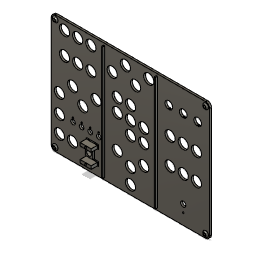
CP-BO Front v3 (Autodesk Fusion 360 design; units mm, degrees)
Autodesk Fusion 360 part; units mm, degrees
note: some values were not read from the file. Set by a fixed rule: which sketch regions a step uses.
sketch "Esquisse1" plane through (0, 0, 0) normal (0, 0, 1) x (1, 0, 0)
  line L0 (10, 0) -> (255, 0)
  line L1 (265, 10) -> (265, 190)
  line L2 (255, 200) -> (10, 200)
  line L3 (0, 190) -> (0, 10)
  arc A0 (10, 200) -> (0, 190) centre (10, 190) ccw
  arc A1 (265, 190) -> (255, 200) centre (255, 190) ccw
  arc A2 (255, 0) -> (265, 10) centre (255, 10) ccw
  arc A3 (0, 10) -> (10, 0) centre (10, 10) ccw
  line L4 (3.6, 190) -> (3.6, 10)
  arc A4 (3.6, 10) -> (10, 3.6) centre (10, 10) ccw
  line L5 (10, 3.6) -> (255, 3.6)
  arc A5 (255, 3.6) -> (261.4, 10) centre (255, 10) ccw
  line L6 (261.4, 10) -> (261.4, 190)
  arc A6 (261.4, 190) -> (255, 196.4) centre (255, 190) ccw
  line L7 (255, 196.4) -> (10, 196.4)
  arc A7 (10, 196.4) -> (3.6, 190) centre (10, 190) ccw
  circle A8 centre (10, 190) radius 1.6
  circle A9 centre (10, 190) radius 2.6
  circle A10 centre (10, 190) radius 3.5
  circle A11 centre (255, 190) radius 1.6
  circle A12 centre (255, 190) radius 2.6
  circle A13 centre (255, 190) radius 3.5
  circle A14 centre (10, 10) radius 1.6
  circle A15 centre (10, 10) radius 2.6
  circle A16 centre (10, 10) radius 3.5
  circle A17 centre (255, 10) radius 1.6
  circle A18 centre (255, 10) radius 2.6
  circle A19 centre (255, 10) radius 3.5
  point P0 (265, 0)
  point P1 (0, 200)
  dimension "d1" = 265
  dimension "d2" = 200
  dimension "d3" = 10
  dimension "d4" = -3.6
  dimension "d5" = 3.2
  dimension "d6" = 5.2
  dimension "d7" = 7
  dimension "d10" = 245
  dimension "d11" = -180
  constraint horizontal L0
  constraint vertical L1
  constraint horizontal L2
  constraint vertical L3
  constraint coincident P1 L2
  constraint coincident P1 L3
  constraint tangent L2 A0
  constraint tangent L3 A0
  constraint tangent L1 A1
  constraint tangent L2 A1
  constraint equal A0 A1
  constraint coincident P0 L0
  constraint coincident P0 L1
  constraint tangent L0 A2
  constraint tangent L1 A2
  constraint equal A0 A2
  constraint coincident origin L0
  constraint coincident origin L3
  constraint tangent L0 A3
  constraint tangent L3 A3
  constraint equal A0 A3
  constraint concentric A0 A8
  constraint concentric A0 A9
  constraint concentric A0 A10
  measures "d1" distance of origin P0
  measures "d2" distance of origin P1
  measures "d3" radius of A0
  measures "d5" diameter of A8
  measures "d6" diameter of A9
  measures "d7" diameter of A10
extrude "Extrusion1" add sketch "Esquisse1" along normal blind 3 contours L4 A4 L5 A5 L6 A6 L7 A7
extrude "Extrusion2" add sketch "Esquisse1" along normal blind 3 and the other way blind -2 contours A9 | A10 | A12 | A13 | A15 | A16 | A18 | A19
extrude "Extrusion3" add sketch "Esquisse1" along normal blind 5 and the other way blind -2 contours A9 | A12 | A15 | A18
fillet "Congé1" radius 2 4 edges at (252.5759, 10.9402, 3) (7.5759, 10.9402, 3) (7.5759, 190.9402, 3) (252.5759, 190.9402, 3)
sketch "Esquisse2" plane through (0, 0, 3) normal (0, 0, 1) x (1, 0, 0)
  circle A0 centre (10, 190) radius 4.6
  circle A1 centre (255, 10) radius 4.6
  arc A2 (10, 196.4) -> (3.6, 190) centre (10, 190) ccw
  line L0 (3.6, 190) -> (3.6, 10)
  arc A3 (3.6, 10) -> (10, 3.6) centre (10, 10) ccw
  line L1 (10, 3.6) -> (255, 3.6)
  arc A4 (255, 3.6) -> (261.4, 10) centre (255, 10) ccw
  line L2 (261.4, 10) -> (261.4, 190)
  arc A5 (261.4, 190) -> (255, 196.4) centre (255, 190) ccw
  line L3 (255, 196.4) -> (10, 196.4)
  circle A6 centre (10, 10) radius 4.6
  circle A7 centre (255, 190) radius 4.6
  line L4 (89.5333, 196.4) -> (89.5333, 3.6) construction
  line L5 (175.4667, 196.4) -> (175.4667, 3.6) construction
  line L6 (175.4667, 33.6) -> (261.4, 33.6) construction
  line L7 (175.4667, 76.2) -> (261.4, 76.2) construction
  line L8 (175.4667, 118.8) -> (261.4, 118.8) construction
  line L9 (175.4667, 161.4) -> (261.4, 161.4) construction
  line L10 (196.95, 196.4) -> (196.95, 3.6) construction
  line L11 (218.4333, 196.4) -> (218.4333, 3.6) construction
  line L12 (239.9167, 196.4) -> (239.9167, 3.6) construction
  circle A8 centre (218.4333, 33.6) radius 4.2
  circle A9 centre (196.95, 76.2) radius 8.3
  circle A10 centre (218.4333, 76.2) radius 8.3
  circle A11 centre (239.9167, 76.2) radius 8.3
  circle A12 centre (196.95, 118.8) radius 8.3
  circle A13 centre (218.4333, 118.8) radius 8.3
  circle A14 centre (239.9167, 118.8) radius 8.3
  line L13 (188.65, 100) -> (188.65, 105) construction
  line L14 (188.65, 105) -> (188.65, 196.4) construction
  line L15 (248.2167, 100) -> (248.2167, 196.4) construction
  circle A15 centre (218.4333, 161.4) radius 6.25
  circle A16 centre (194.9, 161.4) radius 6.25
  circle A17 centre (241.9667, 161.4) radius 6.25
  line L16 (89.5333, 18) -> (175.4667, 18) construction
  line L17 (89.5333, 55.2106) -> (175.4667, 55.2106) construction
  line L18 (111.0167, 196.4) -> (111.0167, 3.6) construction
  line L19 (132.5, 196.4) -> (132.5, 3.6) construction
  line L20 (153.9833, 196.4) -> (153.9833, 3.6) construction
  circle A18 centre (111.0167, 55.2106) radius 8.3
  circle A19 centre (153.9833, 55.2106) radius 8.3
  circle A20 centre (132.5, 18) radius 8.3
  circle A21 centre (132.5, 42.8106) radius 8.3
  line L21 (89.5333, 108.6053) -> (175.4667, 108.6053) construction
  line L22 (89.5333, 87.1223) -> (175.4667, 87.1223) construction
  line L23 (89.5333, 130.0883) -> (175.4667, 130.0883) construction
  circle A22 centre (132.5, 108.6053) radius 8.3
  circle A23 centre (153.9833, 108.6053) radius 8.3
  circle A24 centre (111.0167, 108.6053) radius 8.3
  circle A25 centre (132.5, 130.0883) radius 8.3
  circle A26 centre (111.0167, 130.0883) radius 8.3
  circle A27 centre (132.5, 87.1223) radius 8.3
  circle A28 centre (153.9833, 87.1223) radius 8.3
  line L24 (89.5333, 182) -> (175.4667, 182) construction
  line L25 (89.5333, 162) -> (175.4667, 162) construction
  circle A29 centre (162.2833, 182) radius 8.3
  circle A30 centre (140.8, 162) radius 8.3
  circle A31 centre (124.2, 182) radius 8.3
  circle A32 centre (102.7167, 162) radius 8.3
  line L26 (68.05, 196.4) -> (68.05, 3.6) construction
  line L27 (46.5667, 196.4) -> (46.5667, 3.6) construction
  line L28 (25.0833, 196.4) -> (25.0833, 3.6) construction
  line L29 (89.5333, 182) -> (3.6, 182) construction
  line L30 (89.5333, 145.8) -> (3.6, 145.8) construction
  line L31 (89.5333, 109.6) -> (3.6, 109.6) construction
  line L32 (89.5333, 89.6) -> (3.6, 89.6) construction
  line L33 (89.5333, 59.6) -> (3.6, 59.6) construction
  line L34 (89.5333, 31.6) -> (3.6, 31.6) construction
  circle A33 centre (25.0833, 182) radius 8.3
  circle A34 centre (46.5667, 182) radius 8.3
  circle A35 centre (68.05, 182) radius 8.3
  circle A36 centre (25.0833, 145.8) radius 8.3
  circle A37 centre (46.5667, 145.8) radius 8.3
  circle A38 centre (68.05, 145.8) radius 8.3
  circle A39 centre (76.35, 109.6) radius 8.3
  circle A40 centre (38.2667, 109.6) radius 8.3
  circle A41 centre (54.8667, 89.6) radius 8.3
  circle A42 centre (16.7833, 89.6) radius 8.3
  line L35 (16.7833, 108.886) -> (16.7833, 3.6) construction
  circle A43 centre (16.7833, 59.6) radius 8.3
  circle A44 centre (16.7833, 31.6) radius 8.3
  line L36 (39.0375, 69) -> (39.0375, 49) construction
  line L37 (52.9917, 69) -> (52.9917, 49) construction
  line L38 (66.9458, 69) -> (66.9458, 49) construction
  line L39 (80.9, 69) -> (80.9, 48.7369) construction
  circle A45 centre (39.0375, 59.6) radius 3.75
  circle A46 centre (52.9917, 59.6) radius 3.75
  circle A47 centre (66.9458, 59.6) radius 3.75
  circle A48 centre (80.9, 59.6) radius 3.75
  line L40 (84.65, 126.0158) -> (84.65, 39.0422) construction
  line L41 (194.9, 171) -> (194.9, 151) construction
  line L42 (241.9667, 172) -> (241.9667, 151) construction
  line L43 (194.2, 156.2) -> (195.6, 156.2)
  line L44 (195.6, 156.2) -> (195.6, 155.15)
  line L45 (195.6, 155.15) -> (194.2, 155.15)
  line L46 (194.2, 155.15) -> (194.2, 156.2)
  line L47 (217.7333, 156.2) -> (219.1333, 156.2)
  line L48 (219.1333, 156.2) -> (219.1333, 155.15)
  line L49 (219.1333, 155.15) -> (217.7333, 155.15)
  line L50 (217.7333, 155.15) -> (217.7333, 156.2)
  line L51 (241.2667, 156.2) -> (242.6667, 156.2)
  line L52 (242.6667, 156.2) -> (242.6667, 155.15)
  line L53 (242.6667, 155.15) -> (241.2667, 155.15)
  line L54 (241.2667, 155.15) -> (241.2667, 156.2)
  circle A49 centre (218.4333, 21.6) radius 1.3
  line L55 (87, 65.6) -> (36, 65.6) construction
  circle A50 centre (39.0375, 65.6) radius 1.25
  circle A51 centre (52.9917, 65.6) radius 1.25
  circle A52 centre (66.9458, 65.6) radius 1.25
  circle A53 centre (80.9, 65.6) radius 1.25
  circle A54 centre (68.05, 31.6) radius 3.95
  line L56 (38.0624, 123.6693) -> (38.0624, 15) construction
  circle A55 centre (38.0624, 31.6) radius 8.3
  line L57 (88.5333, 192.8) -> (90.5333, 192.8)
  line L58 (90.5333, 192.8) -> (90.5333, 7.2)
  line L59 (90.5333, 7.2) -> (88.5333, 7.2)
  line L60 (88.5333, 7.2) -> (88.5333, 192.8)
  line L61 (174.4667, 192.8) -> (176.4667, 192.8)
  line L62 (176.4667, 192.8) -> (176.4667, 7.2)
  line L63 (176.4667, 7.2) -> (174.4667, 7.2)
  line L64 (174.4667, 7.2) -> (174.4667, 192.8)
  line L65 (57.05, 42.6) -> (84.05, 42.6) construction
  line L66 (84.05, 42.6) -> (84.05, 23.6) construction
  line L67 (84.05, 23.6) -> (57.05, 23.6) construction
  line L68 (57.05, 23.6) -> (57.05, 42.6) construction
  line L69 (61.55, 42.6) -> (79.55, 42.6)
  line L70 (79.55, 42.6) -> (79.55, 47.6)
  line L71 (79.55, 47.6) -> (61.55, 47.6)
  line L72 (61.55, 47.6) -> (61.55, 42.6)
  line L73 (61.55, 23.6) -> (79.55, 23.6)
  line L74 (79.55, 23.6) -> (79.55, 18.6)
  line L75 (79.55, 18.6) -> (61.55, 18.6)
  line L76 (61.55, 18.6) -> (61.55, 23.6)
  line L77 (70.55, 23.6) -> (70.55, 47.6) construction
  line L78 (61.55, 45.1) -> (79.55, 45.1) construction
  line L79 (61.55, 21.1) -> (79.55, 21.1) construction
  circle A56 centre (70.55, 45.1) radius 1.5
  circle A57 centre (70.55, 21.1) radius 1.5
  line L80 (62.05, 37.6) -> (74.05, 37.6)
  line L81 (74.05, 37.6) -> (74.05, 25.6)
  line L82 (74.05, 25.6) -> (62.05, 25.6)
  line L83 (62.05, 25.6) -> (62.05, 37.6)
  dimension "d24" = 30
  dimension "d27" = 35
  dimension "d29" = 8.4
  dimension "d30" = 16.6
  dimension "d31" = 16.6
  dimension "d32" = 16.6
  dimension "d33" = 16.6
  dimension "d34" = 16.6
  dimension "d35" = 16.6
  dimension "d36" = 12.5
  dimension "d37" = 12.5
  dimension "d38" = 12.5
  dimension "d39" = 14.4
  dimension "d40" = 16.6
  dimension "d41" = 16.6
  dimension "d42" = 16.6
  dimension "d43" = 42.967
  dimension "d44" = 16.6
  dimension "d45" = 12.4
  dimension "d46" = 37.2106
  dimension "d47" = 16.6
  dimension "d48" = 16.6
  dimension "d49" = 16.6
  dimension "d50" = 16.6
  dimension "d51" = 16.6
  dimension "d52" = 16.6
  dimension "d53" = 16.6
  dimension "d54" = 21.483
  dimension "d55" = 21.667
  dimension "d56" = 21.4833
  dimension "d57" = 14.4
  dimension "d58" = 16.6
  dimension "d59" = 16.6
  dimension "d60" = 16.6
  dimension "d61" = 16.6
  dimension "d62" = 20
  dimension "d63" = 16.6
  dimension "d64" = 16.6
  dimension "d65" = 16.6
  dimension "d66" = 14.4
  dimension "d67" = 16.6
  dimension "d68" = 16.6
  dimension "d69" = 16.6
  dimension "d70" = 20
  dimension "d71" = 16.6
  dimension "d72" = 16.6
  dimension "d73" = 16.6
  dimension "d74" = 16.6
  dimension "d75" = 16.6
  dimension "d76" = 16.6
  dimension "d77" = 28
  dimension "d78" = 7.5
  dimension "d79" = 7.5
  dimension "d80" = 7.5
  dimension "d81" = 7.5
  dimension "d84" = 28
  dimension "d86" = 30
  dimension "d87" = 32.6492
  dimension "d88" = 1.4
  dimension "d89" = 1.4
  dimension "d90" = 1.4
  dimension "d91" = 5.2
  dimension "d92" = 5.2
  dimension "d93" = 5.2
  dimension "d94" = 2.6
  dimension "d95" = 12
  dimension "d96" = 2.5
  dimension "d97" = 2.5
  dimension "d98" = 2.5
  dimension "d99" = 2.5
  dimension "d100" = 6
  dimension "d101" = 7.9
  dimension "d102" = 16.6
  dimension "d110" = 2
  dimension "d111" = 2
  dimension "d114" = 3.6
  dimension "d115" = 3.6
  dimension "d116" = 3.6
  dimension "d117" = 3.6
  dimension "d126" = 19
  dimension "d127" = 27
  dimension "d128" = 11
  dimension "d129" = 8
  dimension "d130" = 18
  dimension "d131" = 18
  dimension "d132" = 5
  dimension "d133" = 5
  dimension "d134" = 3
  dimension "d135" = 3
  dimension "d136" = 12
  dimension "d137" = 12
  constraint coincident L3 L4.start
  constraint coincident L1 L4.end
  constraint perpendicular L1 L4
  constraint coincident L3 L5.start
  constraint perpendicular L1 L5
  constraint coincident L5 L6.start
  constraint coincident L2 L6.end
  constraint perpendicular L2 L6
  constraint coincident L5 L7.start
  constraint coincident L2 L7.end
  constraint perpendicular L2 L7
  constraint coincident L5 L8.start
  constraint coincident L2 L8.end
  constraint perpendicular L2 L8
  constraint coincident L5 L9.start
  constraint coincident L2 L9.end
  constraint perpendicular L2 L9
  constraint symmetric L7 L8 L9
  constraint symmetric L6 L7 L8
  constraint coincident L3 L10.start
  constraint coincident L1 L10.end
  constraint perpendicular L1 L10
  constraint coincident L3 L11.start
  constraint coincident L1 L11.end
  constraint perpendicular L1 L11
  constraint coincident L1 L12.end
  constraint perpendicular L1 L12
  constraint symmetric L10 L11 L12
  constraint symmetric L5 L10 L11
  constraint coincident L11 A8.centre
  constraint coincident L6 A8.centre
  constraint coincident L7 A9.centre
  constraint coincident L10 A9.centre
  constraint midpoint L7 A10.centre
  constraint coincident L12 A11.centre
  constraint coincident L7 A11.centre
  constraint coincident L10 A12.centre
  constraint coincident L8 A12.centre
  constraint midpoint L8 A13.centre
  constraint coincident L8 A14.centre
  constraint coincident L12 A14.centre
  constraint perpendicular L8 L13
  constraint perpendicular L9 L14
  constraint coincident L3 L15.end
  constraint perpendicular L3 L15
  constraint coincident L3 L14.end
  constraint tangent A12 L14
  constraint tangent A14 L15
  constraint midpoint L9 A15.centre
  constraint coincident L9 A16.centre
  constraint coincident L9 A17.centre
  constraint tangent L14 A16
  constraint tangent L15 A17
  constraint coincident L4 L16.start
  constraint coincident L5 L16.end
  constraint perpendicular L5 L16
  constraint coincident L4 L17.start
  constraint coincident L5 L17.end
  constraint perpendicular L5 L17
  constraint coincident L3 L18.start
  constraint coincident L1 L18.end
  constraint perpendicular L1 L18
  constraint coincident L3 L19.start
  constraint perpendicular L16 L19
  constraint coincident L3 L20.start
  constraint coincident L1 L20.end
  constraint perpendicular L1 L20
  constraint coincident L1 L19.end
  constraint symmetric L5 L19 L20
  constraint symmetric L4 L18 L19
  constraint coincident L18 A18.centre
  constraint coincident L17 A18.centre
  constraint coincident L17 A19.centre
  constraint coincident L20 A19.centre
  constraint midpoint L16 A20.centre
  constraint coincident L19 A21.centre
  constraint coincident L4 L21.start
  constraint coincident L5 L21.end
  constraint coincident L4 L22.start
  constraint coincident L5 L22.end
  constraint perpendicular L5 L22
  constraint coincident L4 L23.start
  constraint coincident L5 L23.end
  constraint perpendicular L5 L23
  constraint midpoint L21 A22.centre
  constraint coincident L21 A23.centre
  constraint coincident L20 A23.centre
  constraint coincident L21 A24.centre
  constraint coincident L18 A24.centre
  constraint midpoint L23 A25.centre
  constraint coincident L23 A26.centre
  constraint coincident L18 A26.centre
  constraint midpoint L22 A27.centre
  constraint coincident L20 A28.centre
  constraint coincident L22 A28.centre
  constraint symmetric L21 L22 L23
  constraint coincident L4 L24.start
  constraint coincident L5 L24.end
  constraint perpendicular L5 L24
  constraint coincident L4 L25.start
  constraint perpendicular L20 L25
  constraint coincident L24 A29.centre
  constraint coincident L25 A30.centre
  constraint coincident L24 A31.centre
  constraint coincident L25 A32.centre
  constraint tangent L20 A29
  constraint tangent L18 A32
  constraint symmetric L17 L21 L25
  constraint tangent L19 A30
  constraint tangent L19 A31
  constraint coincident L3 L26.start
  constraint coincident L1 L26.end
  constraint perpendicular L1 L26
  constraint coincident L3 L27.start
  constraint coincident L1 L27.end
  constraint perpendicular L1 L27
  constraint coincident L3 L28.start
  constraint coincident L1 L28.end
  constraint perpendicular L1 L28
  constraint symmetric L26 L27 L28
  constraint coincident L0 L29.end
  constraint perpendicular L0 L29
  constraint coincident L4 L30.start
  constraint coincident L0 L30.end
  constraint perpendicular L0 L30
  constraint coincident L4 L31.start
  constraint coincident L0 L31.end
  constraint perpendicular L0 L31
  constraint coincident L4 L32.start
  constraint coincident L0 L32.end
  constraint perpendicular L0 L32
  constraint coincident L4 L33.start
  constraint coincident L0 L33.end
  constraint perpendicular L0 L33
  constraint coincident L4 L34.start
  constraint coincident L0 L34.end
  constraint perpendicular L0 L34
  constraint coincident L29 A33.centre
  constraint coincident L28 A33.centre
  constraint midpoint L29 A34.centre
  constraint coincident L29 A35.centre
  constraint coincident L26 A35.centre
  constraint coincident L30 A36.centre
  constraint coincident L28 A36.centre
  constraint midpoint L30 A37.centre
  constraint coincident L30 A38.centre
  constraint coincident L26 A38.centre
  constraint coincident L31 A40.centre
  constraint coincident L32 A41.centre
  constraint coincident L32 A42.centre
  constraint tangent L27 A40
  constraint tangent L26 A39
  constraint tangent L27 A41
  constraint tangent L28 A42
  constraint coincident L1 L35.end
  constraint perpendicular L1 L35
  constraint coincident A42.centre L35
  constraint coincident L35 A43.centre
  constraint coincident L33 A43.centre
  constraint coincident L35 A44.centre
  constraint coincident L34 A44.centre
  constraint perpendicular L33 L36
  constraint perpendicular L33 L37
  constraint perpendicular L33 L38
  constraint perpendicular L33 L39
  constraint symmetric L36 L37 L38
  constraint coincident L36 A45.centre
  constraint coincident L33 A45.centre
  constraint coincident L33 A46.centre
  constraint coincident L33 A47.centre
  constraint coincident L39 A48.centre
  constraint coincident L33 A48.centre
  constraint coincident L37 A46.centre
  constraint coincident L38 A47.centre
  constraint coincident L31 A39.centre
  constraint tangent A48 L40
  constraint tangent A39 L40
  constraint parallel L4 L40
  constraint symmetric L29 L30 L31
  constraint parallel L10 L41
  constraint perpendicular L9 L42
  constraint coincident A17.centre L42
  constraint coincident A16.centre L41
  constraint horizontal L43
  constraint vertical L44
  constraint horizontal L45
  constraint vertical L46
  constraint horizontal L47
  constraint vertical L48
  constraint horizontal L49
  constraint vertical L50
  constraint horizontal L51
  constraint vertical L52
  constraint horizontal L53
  constraint vertical L54
  constraint symmetric L41 L44 L46
  constraint symmetric L11 L48 L50
  constraint symmetric L42 L52 L54
  constraint tangent A16 L45
  constraint tangent A15 L49
  constraint tangent A17 L53
  constraint coincident L11 A49.centre
  constraint perpendicular L36 L55
  constraint coincident L55 A50.centre
  constraint coincident L55 A51.centre
  constraint coincident L55 A52.centre
  constraint coincident L55 A53.centre
  constraint coincident L36 A50.centre
  constraint coincident L37 A51.centre
  constraint coincident L38 A52.centre
  constraint coincident L39 A53.centre
  constraint coincident L34 A54.centre
  constraint coincident L26 A54.centre
  constraint perpendicular L34 L56
  constraint coincident L34 A55.centre
  constraint coincident L56 A55.centre
  constraint horizontal L57
  constraint vertical L58
  constraint horizontal L59
  constraint vertical L60
  constraint horizontal L61
  constraint vertical L62
  constraint horizontal L63
  constraint vertical L64
  constraint symmetric L4 L58 L60
  constraint symmetric L5 L62 L64
  constraint coincident L1 L5.end
  constraint horizontal L65
  constraint vertical L66
  constraint horizontal L67
  constraint vertical L68
  constraint horizontal L69
  constraint vertical L70
  constraint horizontal L71
  constraint vertical L72
  constraint coincident L65 L69.start
  constraint horizontal L73
  constraint vertical L74
  constraint horizontal L75
  constraint vertical L76
  constraint coincident L67 L73.start
  constraint midpoint L67 L77.start
  constraint coincident L71 L77.end
  constraint perpendicular L71 L77
  constraint symmetric L70 L72 L77
  constraint symmetric L74 L76 L77
  constraint midpoint L72 L78.start
  constraint midpoint L70 L78.end
  constraint midpoint L76 L79.start
  constraint midpoint L74 L79.end
  constraint midpoint L78 A56.centre
  constraint midpoint L79 A57.centre
  constraint horizontal L80
  constraint vertical L81
  constraint horizontal L82
  constraint vertical L83
  constraint symmetric L34 L80 L82
  constraint symmetric L26 L81 L83
  measures "d24" distance of L1 L6
  measures "d27" distance of L3 L9
  measures "d29" diameter of A8
  measures "d30" diameter of A9
  measures "d31" diameter of A10
  measures "d32" diameter of A11
  measures "d33" diameter of A12
  measures "d34" diameter of A13
  measures "d35" diameter of A14
  measures "d36" diameter of A15
  measures "d37" diameter of A16
  measures "d38" diameter of A17
  measures "d39" distance of L1 L16
  measures "d40" diameter of A18
  measures "d41" diameter of A19
  measures "d42" diameter of A20
  measures "d43" distance of A19.centre A20.centre
  measures "d44" diameter of A21
  measures "d45" distance of L17 A21.centre
  measures "d46" distance of L16 L17
  measures "d47" diameter of A22
  measures "d48" diameter of A23
  measures "d49" diameter of A24
  measures "d50" diameter of A25
  measures "d51" diameter of A26
  measures "d52" diameter of A27
  measures "d53" diameter of A28
  measures "d54" distance of L21 L22
  measures "d56" distance of L19 L20
  measures "d57" distance of L3 L24
  measures "d58" diameter of A29
  measures "d59" diameter of A30
  measures "d60" diameter of A31
  measures "d61" diameter of A32
  measures "d62" distance of L24 L25
  measures "d63" diameter of A33
  measures "d64" diameter of A34
  measures "d65" diameter of A35
  measures "d66" distance of L3 L29
  measures "d67" diameter of A36
  measures "d68" diameter of A37
  measures "d69" diameter of A38
  measures "d70" distance of L31 L32
  measures "d71" diameter of A39
  measures "d72" diameter of A40
  measures "d73" diameter of A41
  measures "d74" diameter of A42
  measures "d75" diameter of A43
  measures "d76" diameter of A44
  measures "d77" distance of L1 L34
  measures "d78" diameter of A45
  measures "d79" diameter of A46
  measures "d80" diameter of A47
  measures "d81" diameter of A48
  measures "d84" distance of L33 L34
  measures "d86" distance of L32 L33
  measures "d88" distance of L44 L46
  measures "d89" distance of L48 L50
  measures "d90" distance of L52 L54
  measures "d91" distance of L9 L51
  measures "d92" distance of L9 L47
  measures "d93" distance of L9 L43
  measures "d94" diameter of A49
  measures "d95" distance of A8.centre A49.centre
  measures "d96" diameter of A50
  measures "d97" diameter of A51
  measures "d98" diameter of A52
  measures "d99" diameter of A53
  measures "d100" distance of L33 L55
  measures "d101" diameter of A54
  measures "d102" diameter of A55
  measures "d110" distance of L62 L64
  measures "d111" distance of L58 L60
  measures "d114" distance of L1 L59
  measures "d115" distance of L1 L63
  measures "d116" distance of L3 L57
  measures "d117" distance of L3 L61
  measures "d126" distance of L65 L67
  measures "d127" distance of L66 L68
  measures "d128" distance of A54.centre L68
  measures "d129" distance of A54.centre L67
  measures "d130" distance of L70 L72
  measures "d131" distance of L74 L76
  measures "d132" distance of L67 L75
  measures "d133" distance of L69 L71
  measures "d134" diameter of A56
  measures "d135" diameter of A57
  measures "d136" distance of L81 L83
  measures "d137" distance of L80 L82
extrude "Trous" cut sketch "Esquisse2" against normal blind 3 contours A8 | A9 | A10 | A11 | A12 | A13 | A14 | A15 L47 L48 L50 | A16 L43 L44 L46 | A17 L51 L52 L54 | A18 | A19 | A20 | A21 | A22 | A23 | A24 | A25 | A26 | A27 | A28 | A29 | A30 | A31 | A32 | A33 | A34 | A35 | A36 | A37 | A38 | A39 | A40 | A41 | A42 | A43 | A44 | A45 | A46 | A47 | A48 | A54 | A55 picked at (218.3053, 160.0127) picked at (194.7719, 160.0127) picked at (241.8386, 160.0127)
extrude "Extrusion5" cut sketch "Esquisse2" against normal blind 2 contours A49
extrude "Extrusion6" cut sketch "Esquisse2" against normal blind 1.5 contours A50 | A51 | A52 | A53
extrude "Extrusion8" add sketch "Esquisse2" along normal blind 3 contours L57 L58 L59 L60 | L61 L62 L63 L64
extrude "Extrusion9" add sketch "Esquisse2" along normal blind 3 contours L80 L81 L82 L83
extrude "Extrusion10" add sketch "Esquisse2" along normal blind 11 contours L69 L70 L71 L72 | L73 L74 L75 L76
fillet "Congé2" radius 1 8 edges at (70.55, 18.6, 3) (79.55, 21.1, 3) (70.55, 42.6, 3) (79.55, 45.1, 3) (70.55, 47.6, 3) (61.55, 45.1, 3) (70.55, 23.6, 3) (61.55, 21.1, 3)
